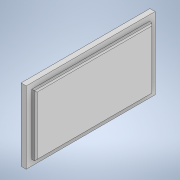
# Autodesk Inventor part: gehaeuse_deckel
Saved by Autodesk Inventor 2020 (Build 240168000, 168)
## iProperties
Created: 2020-05-23
Part Number: gehaeuse_deckel
Material: Generisch
Document SubType Name: Modeling
Designer: chris
Density: 1 g/cm^3
Appearance: Vorgabe
Author: chris
Autodesk Inventor part; units mm, degrees
ref_plane "YZ Plane" through (0, 0, 0) normal (1, 0, 0) x (0, 1, 0)
ref_plane "XZ Plane" through (0, 0, 0) normal (0, 1, 0) x (-1, 0, 0)
ref_plane "XY Plane" through (0, 0, 0) normal (0, 0, 1) x (1, 0, 0)
sketch "Skizze1" plane through (0, 0, 0) normal (1, 0, 0) x (0, 1, 0)
  line L0 (0, 0) -> (28, 0)
  line L1 (28, 0) -> (28, -50)
  line L2 (28, -50) -> (0, -50)
  line L3 (0, -50) -> (0, 0)
  dimension "d0" = 50
  dimension "d1" = 28
  constraints: 8 end point, 2 parallel, 1 horizontal, 1 perpendicular
  measures "d0" distance of L2.end L0.start
  measures "d1" distance of L0.start L0.end
extrude "Extrusion1" add sketch "Skizze1" along normal blind 2
sketch "Skizze2" plane through (2, 0, 0) normal (1, 0, 0) x (0, 0, -1)
  line L0 (2.2, 25.8) -> (47.8, 25.8)
  line L1 (47.8, 25.8) -> (47.8, 2.2)
  line L2 (47.8, 2.2) -> (2.2, 2.2)
  line L3 (2.2, 2.2) -> (2.2, 25.8)
  line L4 (0, 28) -> (0, 0) projected
  line L5 (0, 0) -> (50, 0) projected
  dimension "d4" = 45.6
  dimension "d5" = 23.6
  dimension "d6" = 2.2
  dimension "d7" = 2.2
  constraints: 8 end point, 2 parallel, 1 horizontal, 1 perpendicular
  measures "d4" distance between parallel lines of L1 L3
  measures "d5" distance between parallel lines of L2 L0
  measures "d6" distance between parallel lines of L4 L3
  measures "d7" distance between parallel lines of L5 L2
extrude "Extrusion2" add sketch "Skizze2" along normal blind 1.5
chamfer "Fase1" distance 0.5 angle 45 4 edges at (3.5, 2.2, -25) (3.5, 14, -2.2) (3.5, 14, -47.8) (3.5, 25.8, -25)
